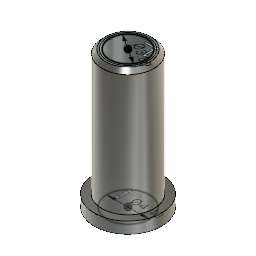
Q_11 (Merc) (Autodesk Fusion 360 design; units mm, degrees)
Autodesk Fusion 360 part; units mm, degrees
sketch "Sketch1" plane through (0, 0, 0) normal (0, 0, 1) x (1, 0, 0)
  circle A0 centre (0, 0) radius 3.5
  dimension "d1" = 7
  constraint coincident A0.centre origin
  measures "d1" diameter of A0
extrude "Extrude1" add sketch "Sketch1" along normal blind 1.2
sketch "Sketch2" plane through (0, 0, 1.2) normal (0, 0, 1) x (-1, 0, 0)
  circle A0 centre (0, 0) radius 3.5
  circle A1 centre (0, 0) radius 2.7
  dimension "d4" = 5.4
  constraint coincident A0.centre A1.centre
  measures "d4" diameter of A1
extrude "Extrude2" add sketch "Sketch2" along normal blind 13 contours A1
chamfer "Chamfer1" distance 0.4 angle 45 1 edges at (2.5173, 0.9764, 14.2)
sketch "Sketch3" plane through (0, 0, 14.2) normal (0, 0, 1) x (-1, 0, 0)
  circle A0 centre (0, 0) radius 2.3
  circle A1 centre (0, 0) radius 1.9
  dimension "d8" = 3.8
  constraint coincident A0.centre A1.centre
  measures "d8" diameter of A1
hole "Hole1" at (0, 0, 14.2) direction (0, 0, -1) diameter 4.2 depth 11 tip angle 180
sketch "Sketch4" plane through (0, 0, 0) normal (0, 0, -1) x (1, 0, 0)
  circle A0 centre (0, 0) radius 3.5
  circle A1 centre (0, 0) radius 2.2
  dimension "d12" = 4.4
  constraint coincident A0.centre A1.centre
  measures "d12" diameter of A1
hole "Hole2" at (0, 0, 0) direction (0, 0, 1) diameter 4.4 depth 3.2 tip angle 180
